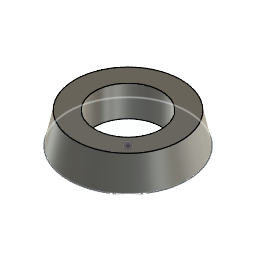
rond-bouton (Autodesk Fusion 360 design; units mm, degrees)
Autodesk Fusion 360 part; units mm, degrees
sketch "Esquisse1" plane through (0, 0, 0) normal (0, 0, 1) x (1, 0, 0)
  circle A0 centre (0, 0) radius 6.75
  dimension "d1" = 13.5
  constraint coincident A0.centre origin
  measures "d1" diameter of A0
extrude "Extrusion1" add sketch "Esquisse1" along normal blind 3.5 makes body 1
sketch "Esquisse2" plane through (0, 0, 3.5) normal (0, 0, 1) x (-1, 0, 0)
  circle A0 centre (0, 0) radius 6.75
  circle A1 centre (0, 0) radius 6
  dimension "d4" = 12
  constraint concentric A0 A1
  measures "d4" diameter of A1
loft "Lissage1" add profiles "Esquisse1", "Esquisse2" section 1 section 2 contours A1 separate body makes body 2
sketch "Esquisse3" plane through (0, 0, 0) normal (0, 0, 1) x (1, 0, 0)
  circle A0 centre (0, 0) radius 3.375
  dimension "d5" = 6.75
  constraint coincident A0.centre origin
  measures "d5" diameter of A0
extrude "Extrusion2" cut sketch "Esquisse3" along normal blind 33 bodies 2
sketch "Esquisse4" plane through (0, 0, 0) normal (0, 0, 1) x (1, 0, 0)
  circle A0 centre (0, 0) radius 3.75
  dimension "d8" = 7.5
  constraint coincident A0.centre origin
  measures "d8" diameter of A0
extrude "Extrusion3" cut sketch "Esquisse4" along normal blind 23 bodies 2
hidden bodies 1
